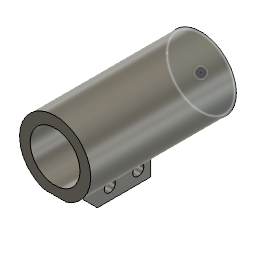
Firing Nozzle (Autodesk Fusion 360 design; units mm, degrees)
part number: 2026-08-23-02-59-21-241
Autodesk Fusion 360 part; units mm, degrees
sketch "Sketch1" plane through (0, 0, 0) normal (0, 0, 1) x (1, 0, 0)
  circle A0 centre (0, 0) radius 7
  circle A1 centre (0, 0) radius 10
  line L0 (0, 0) -> (0, -9.5) construction
  line L1 (-18, -9.5) -> (18, -9.5)
  line L2 (-1.9, -9.5) -> (1.9, -9.5)
  line L3 (-1.9, -9.5) -> (-1.9, -16.5)
  line L4 (1.9, -9.5) -> (1.9, -16.5)
  line L5 (-1.9, -16.5) -> (1.9, -16.5)
  dimension "d1" = 14
  dimension "d2" = 20
  dimension "d3" = 9.5
  dimension "d9" = 36
  dimension "d12" = 3.8
  dimension "d13" = 7
  dimension "d14" = 7
  constraint coincident A0.centre A1.centre
  constraint concentric A0 A1
  constraint vertical L0
  constraint midpoint L0.end L1
  constraint perpendicular L0 L1
  constraint midpoint L0.end L2
  constraint perpendicular L0 L2
  constraint vertical L3
  constraint vertical L4
  measures "d1" diameter of A0
  measures "d2" diameter of A1
  measures "d3" distance of A0.centre L0.end
  measures "d9" distance of L1.start L1.end
  measures "d12" distance of L2.start L2.end
  measures "d13" distance of L2.start L3.end
  measures "d14" distance of L2.end L4.end
extrude "Extrude3" add sketch "Sketch1" along normal blind 25 contours A1 L1 L2
extrude "Extrude4" add sketch "Sketch1" along normal blind 22 contours A1 L1 L2 L3 L4 | A1 L3 L4 L5
sketch "Sketch3" plane through (1.9, 0, 0) normal (1, 0, 0) x (0, 0, -1)
  line L0 (0, -16.5) -> (0, -9.5)
  line L1 (0, -9.5) -> (-22, -9.5)
  line L2 (-22, -9.5) -> (-22, -16.5)
  line L3 (-22, -16.5) -> (0, -16.5)
  line L4 (-22, -9.5) -> (-15, -16.5)
  line L5 (0, -9.5) -> (0, -16.5)
  dimension "d17" = 15
  constraint coincident L1.end L2.start
  constraint coincident L3 L4.end
  measures "d17" distance of L4.end L5
extrude "Extrude5" cut sketch "Sketch3" against normal blind 3.8 contours L2 L3 L4
hole "Hole1" at (1.9, -13, 11.5) direction (-1, 0, 0) diameter 3.1 depth 3.8 tip angle 180
hole "Hole2" at (1.9, -13, 3.5) direction (-1, 0, 0) diameter 3.1 depth 3.8 tip angle 180
extrude "Extrude6" add sketch "Sketch1" against normal blind 16 contours A1 L1 L2
sketch "Sketch4" plane through (0, 0, -16) normal (0, 0, -1) x (-1, 0, 0)
  circle A0 centre (0, 0) radius 7
  line L0 (-3.1225, -9.5) -> (3.1225, -9.5)
  arc A1 (3.1225, -9.5) -> (-3.1225, -9.5) centre (0, 0) ccw
  circle A2 centre (0, 0) radius 9.5
  dimension "d32" = 19
  constraint coincident A0.centre A1.centre
  measures "d32" diameter of A2
ref_plane "WorkPlane1" through (0, 0, -8) normal (0, 0, 1) x (1, 0, 0)
chamfer "Chamfer1" distance 3 angle 45 1 edges at (-6.5263, -2.5313, -16)
